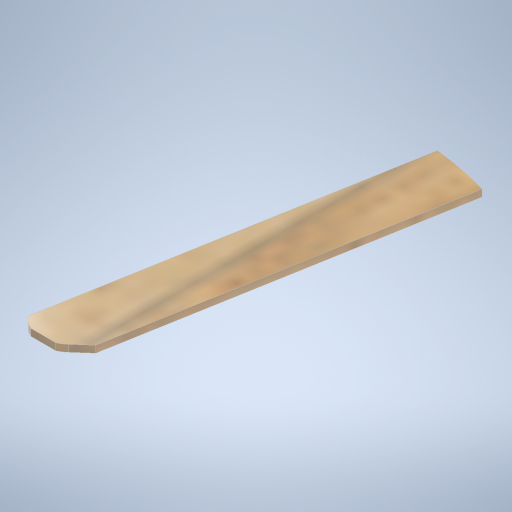
# Autodesk Inventor part: dish_under
Saved by Autodesk Inventor 2024.1 (Build 281209000, 209)
## iProperties
Created: 2025-09-27
Part Number: dish_under
Material: 木材 (カエデ材)
Document SubType Name: Modeling
Designer: hibik
Density: 0.67 g/cm^3
Appearance: ナチュラル カエデ材 - 光沢 濃い着色
Author: hibik
Autodesk Inventor part; units mm, degrees
ref_plane "YZ Plane" through (0, 0, 0) normal (1, 0, 0) x (0, 1, 0)
ref_plane "XZ Plane" through (0, 0, 0) normal (0, 1, 0) x (-1, 0, 0)
ref_plane "XY Plane" through (0, 0, 0) normal (0, 0, 1) x (1, 0, 0)
sketch "スケッチ1" plane through (0, 0, 0) normal (0, 1, 0) x (-1, 0, 0)
  circle A0 centre (0, 0) radius 11
  line L0 (11, 10) -> (-11, 10)
  line L1 (-11, 10) -> (-11, -10)
  line L2 (-11, -10) -> (11, -10)
  line L3 (11, -10) -> (11, 10)
  line L4 (11, -10) -> (-11, -10)
  line L5 (-11, -10) -> (-11, -110)
  line L6 (-11, -110) -> (11, -110) construction
  line L7 (11, -110) -> (11, -10) construction
  arc A1 (-34.6127, -115.6757) -> (-13.3752, -120) centre (0, 0) ccw
  circle A2 centre (22, 0) radius 11
  circle A3 centre (-22, 0) radius 11
  line L8 (46.542, 0) -> (-48.2519, 0) projected
  line L9 (0, 0) -> (-13.7873, 2.4311)
  line L10 (-13.7873, 2.4311) -> (-34.6127, -115.6757)
  line L11 (22, 0) -> (8.2127, 2.4311)
  line L12 (8.2127, 2.4311) -> (-13.3752, -120)
  line L13 (8.2127, 2.4311) -> (8.9192, 6.438)
  line L14 (-13.7873, 2.4311) -> (-7.33, 8.2019)
  point P0 (11, 0)
  point P1 (11, 0)
  point P2 (4.5826, 10)
  point P3 (-4.5826, 10)
  point P4 (-11, 0)
  point P5 (-11, 0)
  point P6 (-11, 0)
  point P7 (4.5826, -10)
  point P8 (11, 0)
  point P9 (-11, 0)
  point P10 (-4.5826, -10)
  point P11 (4.5826, -10)
  point P12 (-4.5826, -10)
  point P13 (6.1794, -9.1003)
  point P14 (7.784, 0)
  point P15 (10.822, 1.971)
  point P16 (-14.216, 0)
  point P17 (11, 1.9396)
  dimension "d0" = 22
  dimension "d1" = 20
  dimension "d2" = 100
  dimension "d13" = 10
  dimension "d14" = 14
  dimension "d15" = 10
  constraints: 28 end point, 7 point on circle, 6 parallel, 4 horizontal alignment, 4 perpendicular, 3 tangent, 2 centre point, 2 coincident, 2 collinear, 2 horizontal, 2 midpoint, 7 other
  measures "d0" diameter of A0
  measures "d1" distance of L2.end L0.start
  measures "d2" distance of L5.end L4.end
  measures "d13" angle of L8 L9
  measures "d14" distance from line of point (0, 0) L10
  measures "d15" distance from line of L12.end L6
extrude "押し出し1" add sketch "スケッチ1" along normal blind 2.5 contours L12 L2 A0 | A0 L2 L8 L12 | L8 L9 A0 L0 L13 L12 | L2 L12 L5 A0 | A0 L2 | L8 A0 L9 | L2 L1 A0 | L12 A1 L10 A3 L1 L5 | L1 L9 A0 | A3 L9 L1 | L8 L10 L9 A3 | A3 L10 L8 | L9 L1 L14 A0 | L9 A3 L14 L1 | L9 L14 A3 picked at (-14.6149, -5.4805)
sketch "スケッチ2" plane through (0, 2.5, 0) normal (0, 1, 0) x (1, 0, 0)
  line L0 (33.6474, 115.9601) -> (12.5819, -3.5083)
  line L1 (13.7873, -2.4311) -> (34.6127, 115.6757) projected
  arc A0 (34.6127, 115.6757) -> (13.3752, 120) centre (0, 0) ccw projected
  line L2 (7.33, -8.2019) -> (13.7873, -2.4311) projected
  dimension "d16" = 1
  constraints: 2 end point, 1 parallel, 1 point on circle, 1 point on line
  measures "d16" distance between parallel lines of L1 L0
extrude "押し出し2" cut sketch "スケッチ2" against normal through all
